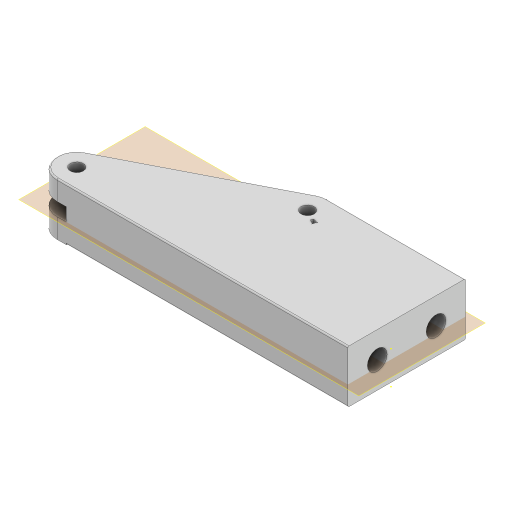
# Autodesk Inventor part: torree3
Saved by Autodesk Inventor 2024 (Build 280153000, 153)
## iProperties
Created: 2024-04-22
Part Number: torree3
Material: Generic
Document SubType Name: Modeling
Designer: alexz
Density: 1 g/cm^3
Appearance: Default
Author: alexz
Autodesk Inventor part; units mm, degrees
ref_plane "YZ Plane" through (0, 0, 0) normal (1, 0, 0) x (0, 1, 0)
sketch "Sketch1" plane through (0, 0, 0) normal (0, 1, 0) x (-1, 0, 0)
  circle A0 centre (238.9, 0) radius 5
  circle A1 centre (122.8, -59.4) radius 5
  line L0 (17.8, 15) -> (17.8, -74.4)
  line L1 (17.8, -74.4) -> (126.4144, -74.4)
  line L2 (17.8, 15) -> (250.6544, 15)
  line L3 (126.4144, -74.4) -> (301.1508, 15)
  line L4 (301.1508, 15) -> (250.6544, 15)
  circle A2 centre (238.9, 0) radius 15
  circle A3 centre (122.8, -59.4) radius 15
  line L5 (108.6104, -54.5363) -> (101.8018, -74.4)
  line L6 (108.6104, -54.5363) -> (129.6086, -54.5363) construction
  line L7 (127.3662, -45.1119) -> (162.016, -56.1852)
  point P0 (0, 0)
  point P1 (122.8, -74.4)
  point P2 (129.6321, -72.7537)
  dimension "d0" = 10
  dimension "d1" = 10
  dimension "d3" = 59.4
  dimension "d4" = 89.4
  dimension "d5" = 15
  dimension "d6" = 15
  dimension "d7" = 15
  dimension "d23" = 108.92
  dimension "d32" = 116.1
  dimension "d33" = 105
  dimension "d34" = 283.3508
  constraints: 16 end point, 4 centre point, 4 tangent, 3 horizontal, 2 coincident, 2 point on circle, 2 point on line, 1 equal length, 1 perpendicular, 1 vertical
  measures "d0" diameter of A0
  measures "d1" diameter of A1
  measures "d3" vertical distance of A0.centre A1.centre
  measures "d4" distance of L0.start L0.end
  measures "d5" distance from line of L2 A0.centre
  measures "d6" distance from line of L3 A0.centre
  measures "d7" distance from line of L3 A1.centre
  measures "d23" angle of L5 L6
  measures "d32" horizontal distance of A1.centre A0.centre
  measures "d33" distance from line of L0 A1.centre
  measures "d34" distance of L0.start L3.end
extrude "Extrusion1" add sketch "Sketch1" along normal blind 40 contours L2 A2 L3 L7 A3 L5 L1 L0 | L2 L4 L3 A2 | A2 | L5 A3 L1 | A3 | L3 A3 L7
fillet "Fillet1" radius 15 1 edges at (-301.1508, 20, 15)
sketch "Sketch2" plane through (-17.8, 0, 15) normal (1, 0, 0) x (0, 0, -1)
  circle A0 centre (67.05, 20) radius 7.5
  line L0 (89.4, 0) -> (89.4, 40) projected
  circle A1 centre (22.35, 20) radius 7.5
  line L1 (0, 0) -> (0, 40) projected
  point P0 (15, 0)
  point P1 (89.4, 20)
  point P2 (0, 20)
  dimension "d12" = 15
  dimension "d13" = 22.35
  dimension "d14" = 15
  dimension "d15" = 22.35
  constraints: 2 centre point, 2 horizontal alignment, 2 midpoint
  measures "d12" diameter of A0
  measures "d13" distance from line of L0 A0.centre
  measures "d14" diameter of A1
  measures "d15" distance from line of L1 A1.centre
extrude "Extrusion2" cut sketch "Sketch2" against normal blind 30
sketch "Sketch4" plane through (0, 40, 0) normal (0, 1, 0) x (1, 0, 0)
  point P0 (0, 0)
extrude "Extrusion5" cut sketch "Sketch1" along normal blind 25 contours L5 A3 L1 | A3 | L3 A3 L7
extrude "Extrusion6" add sketch "Sketch1" along normal blind 15 contours L5 A3 L1 | A3 | L3 A3 L7
fillet "Fillet3" radius 1 10 edges at (-253.4826, 40, 3.5138) (-187.6821, 40, -43.0537) (-126.3138, 40, -73.9826) (-70.3, 40, -74.4) (-128.35, 40, 15) (-253.4826, 0, 3.5138) (-128.35, 0, 15) (-126.3138, 0, -73.9826) (-70.3, 0, -74.4) (-187.6821, 0, -43.0537)
sketch "Sketch5" plane through (0, 0, 0) normal (0, -1, 0) x (1, 0, 0)
  line L0 (-253.9, 15) -> (-231.9, 15)
  line L1 (-238.9, 15) -> (-17.8, 15) projected
  line L2 (-231.9, 15) -> (-206.8624, -33.2406)
  line L3 (-129.6321, -72.7537) -> (-245.7321, -13.3537) projected
  line L4 (-206.8624, -33.2406) -> (-253.9, -9.1748)
  line L5 (-253.9, -9.1748) -> (-253.9, 15)
  arc A0 (-238.9, 15) -> (-245.7321, -13.3537) centre (-238.9, 0) ccw projected
  circle A1 centre (-238.9, 0) radius 5
  point P0 (0, 0)
  dimension "d36" = 22
  dimension "d37" = 117.43
  constraints: 8 end point, 3 point on line, 1 centre point, 1 coincident, 1 collinear, 1 tangent, 1 vertical
  measures "d36" distance of L0.start L0.end
  measures "d37" angle of L0 L2
extrude "Extrusion7" cut sketch "Sketch5" against normal blind 25 contours L0 L2 L3 A0 | A1
extrude "Extrusion8" add sketch "Sketch5" against normal blind 15 contours L0 L2 L3 A0
sketch "Sketch7" plane through (-162.016, 15, -56.1852) normal (-0.4554758, 0, -0.8902482) x (-0.8902482, 0, 0.4554758)
  line L0 (50.3752, 0) -> (50.3752, 10) projected
  point P0 (-118.6434, -15)
  point P1 (50.3752, 5)
  constraints: 1 midpoint
ref_plane "Work Plane1" through (-206.8624, 15, -33.2406) normal (-0.4606646, 0, 0.8875743) x (0, 1, 0)
sketch "Sketch8" plane through (-206.8624, 15, -33.2406) normal (-0.4606646, 0, 0.8875743) x (0, 1, 0)
  circle A0 centre (5, 13.25) radius 13.25
  line L0 (0, 0) -> (10, 0) projected
  point P0 (-15, -198.9185)
  point P1 (5, 0)
  dimension "d45" = 26.5
  constraints: 1 centre point, 1 midpoint, 1 tangent, 1 vertical alignment
  measures "d45" diameter of A0
extrude "Extrusion9" cut sketch "Sketch8" along normal blind 28
ref_plane "Work Plane2" through (-162.016, 0, -56.1852) normal (0.9525404, 0, 0.3044122) x (0, -1, 0)
sketch "Sketch9" plane through (-162.016, 0, -56.1852) normal (0.9525404, 0, 0.3044122) x (0, -1, 0)
  circle A0 centre (-20, 13) radius 13
  line L0 (-25, 0) -> (-15, 0) projected
  point P0 (0, -4.1991)
  point P1 (-20, 0)
  dimension "d49" = 26
  constraints: 1 centre point, 1 midpoint, 1 tangent, 1 vertical alignment
  measures "d49" diameter of A0
extrude "Extrusion10" cut sketch "Sketch9" along normal blind 18
fillet "Fillet4" radius 5 1 edges at (-214.4983, 25, -20.6548)
fillet "Fillet5" radius 5 1 edges at (-214.4983, 15, -20.6548)
fillet "Fillet6" radius 5 1 edges at (-152.6584, 25, -54.2446)
fillet "Fillet7" radius 5 1 edges at (-152.6584, 15, -54.2446)
sketch "Sketch10" plane through (0, 40, 0) normal (0, 1, 0) x (1, 0, 0)
  point P0 (0, 0)
ref_plane "Work Plane3" through (0, 15, 0) normal (0, 1, 0) x (1, 0, 0)
sketch "Sketch13" plane through (0, 15, 0) normal (0, 1, 0) x (1, 0, 0)
  point P0 (0, 0)
sketch "Sketch14" plane through (0, 15, 0) normal (0, 1, 0) x (1, 0, 0)
  spline S0 degree 3 poles (-114.7798, 55.808) (-114.6957, 55.8053) (-114.5275, 55.7999) (-114.2756, 55.7834) (-114.0241, 55.7606) (-113.7735, 55.7305) (-113.5238, 55.6927) (-113.2756, 55.6467) (-113.0291, 55.5918) (-112.8257, 55.5379) (-112.6646, 55.4893) (-112.5447, 55.4498) (-112.4258, 55.4072) (-112.3085, 55.3608) (-112.1925, 55.3108) (-112.08, 55.2535) (-111.964, 55.2034) (-111.8641, 55.17) (-111.7824, 55.1498) (-111.7204, 55.138) (-111.6577, 55.1301) (-111.5947, 55.1265) (-111.5315, 55.1278) (-111.4686, 55.1342) (-111.4066, 55.1463) (-111.3459, 55.1637) (-111.2871, 55.1868) (-111.2306, 55.2152) (-111.1777, 55.2498) (-111.1282, 55.289) (-111.0827, 55.3329) (-111.0303, 55.3989) (-110.9937, 55.4503) (-110.9693, 55.4846) knots 0 0 0 0 0.062504 0.125008 0.187512 0.250015 0.312519 0.375021 0.437524 0.500025 0.531277 0.562529 0.593781 0.625032 0.656283 0.687535 0.718783 0.750029 0.765656 0.781279 0.796902 0.812525 0.82815 0.843776 0.859399 0.875018 0.890637 0.906261 0.921883 0.937503 0.953127 0.968747 1 1 1 1
  spline S1 degree 3 poles (-112.3459, 51.8853) (-112.3409, 51.9272) (-112.3335, 51.9901) (-112.3279, 52.0745) (-112.3322, 52.1378) (-112.3425, 52.2004) (-112.3585, 52.2618) (-112.3814, 52.3209) (-112.4095, 52.3778) (-112.4429, 52.4317) (-112.4808, 52.4824) (-112.5233, 52.5296) (-112.5694, 52.5731) (-112.6186, 52.613) (-112.6705, 52.6493) (-112.7246, 52.6823) (-112.799, 52.7224) (-112.8958, 52.7649) (-113.0157, 52.8059) (-113.138, 52.8392) (-113.2579, 52.8802) (-113.3765, 52.9248) (-113.4935, 52.9733) (-113.6093, 53.0248) (-113.7618, 53.0973) (-113.9494, 53.1944) (-114.1696, 53.3197) (-114.3851, 53.4529) (-114.5962, 53.5931) (-114.8029, 53.7396) (-115.0052, 53.8922) (-115.2036, 54.0498) (-115.3322, 54.1592) (-115.3966, 54.214) knots 0 0 0 0 0.031253 0.046873 0.062497 0.078117 0.093739 0.109363 0.124982 0.140601 0.156224 0.17185 0.187475 0.203098 0.218721 0.234344 0.249971 0.281217 0.312465 0.343717 0.374968 0.406219 0.437471 0.468723 0.499975 0.562476 0.624979 0.687481 0.749985 0.812488 0.874992 0.937496 1 1 1 1
  arc A0 (-114.7798, 55.808) -> (-115.3966, 54.214) centre (-106.6451, 51.7443) ccw
  line L0 (-112.3459, 51.8853) -> (-110.9693, 55.4846)
  point P0 (0, 0)
  point P1 (-111.5946, 55.1273)
  point P2 (-111.6576, 55.1308)
  point P3 (-111.7823, 55.1504)
  point P4 (-111.8435, 55.1655)
  point P5 (-111.9633, 55.2051)
  point P6 (-112.0794, 55.2547)
  point P7 (-112.1931, 55.3095)
  point P8 (-112.3087, 55.3602)
  point P9 (-112.4261, 55.4065)
  point P10 (-112.5448, 55.4493)
  point P11 (-112.6647, 55.4888)
  point P12 (-111.7203, 55.1386)
  point P13 (-114.2756, 55.7824)
  point P14 (-114.0243, 55.7594)
  point P15 (-113.7736, 55.7292)
  point P16 (-113.5241, 55.6913)
  point P17 (-113.2759, 55.6452)
  point P18 (-113.0295, 55.5901)
  point P19 (-112.7856, 55.5253)
  point P20 (-111.5315, 55.1287)
  point P21 (-111.4688, 55.1351)
  point P22 (-111.4068, 55.1472)
  point P23 (-111.3462, 55.1646)
  point P24 (-111.2875, 55.1877)
  point P25 (-111.2312, 55.2162)
  point P26 (-111.1783, 55.2506)
  point P27 (-111.1289, 55.2898)
  point P28 (-111.0837, 55.3339)
  point P29 (-111.0437, 55.3826)
  point P30 (-112.7806, 52.7119)
  point P31 (-112.7249, 52.6819)
  point P32 (-112.6709, 52.6488)
  point P33 (-112.6191, 52.6124)
  point P34 (-112.5699, 52.5725)
  point P35 (-112.5239, 52.529)
  point P36 (-112.4816, 52.4818)
  point P37 (-112.4436, 52.4311)
  point P38 (-112.4104, 52.3773)
  point P39 (-112.3823, 52.3205)
  point P40 (-112.3597, 52.2614)
  point P41 (-112.3332, 52.1377)
  point P42 (-112.3325, 52.0113)
  point P43 (-112.3435, 52.2002)
  point P44 (-112.8964, 52.7633)
  point P45 (-113.0161, 52.8046)
  point P46 (-113.1376, 52.8405)
  point P47 (-113.2577, 52.8808)
  point P48 (-113.4933, 52.9738)
  point P49 (-113.609, 53.0253)
  point P50 (-113.7235, 53.0796)
  point P51 (-112.3293, 52.0745)
  point P52 (-113.3762, 52.9255)
  point P53 (-113.9486, 53.1958)
  point P54 (-114.1688, 53.321)
  point P55 (-114.3844, 53.454)
  point P56 (-114.5955, 53.5941)
  point P57 (-114.8021, 53.7406)
  point P58 (-115.0045, 53.8931)
  point P59 (-115.2027, 54.0509)
  dimension "d59" = -1.594
  dimension "d60" = -3.5993
  dimension "d61" = -3.8105
  dimension "d62" = -3.0506
  constraints: 2 end point, 2 point on circle, 1 centre point, 64 other
  measures "d59" vertical distance of A0.start A0.end
  measures "d60" vertical distance of L0.end L0.start
  measures "d61" horizontal distance of A0.start L0.end
  measures "d62" horizontal distance of L0.start A0.end
extrude "Extrusion11" cut sketch "Sketch14" along normal through all
body "Solid1"
